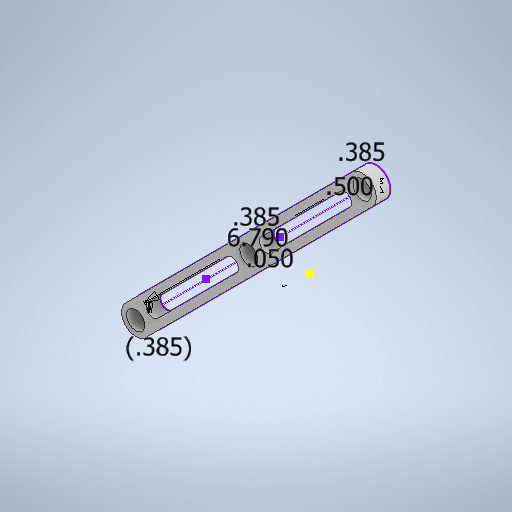
# Autodesk Inventor part: Reg Arm
Saved by Autodesk Inventor 2025.1 (Build 291241000, 241)
## iProperties
Created: 2025-10-25
Part Number: Reg Arm
Material: Generic
Document SubType Name: Modeling
Designer: benja
Density: 1 g/cm^3
Appearance: Default
Author: benja
Autodesk Inventor part; units mm, degrees
ref_plane "YZ Plane" through (0, 0, 0) normal (1, 0, 0) x (0, 1, 0)
ref_plane "XZ Plane" through (0, 0, 0) normal (0, 1, 0) x (-1, 0, 0)
ref_plane "XY Plane" through (0, 0, 0) normal (0, 0, 1) x (1, 0, 0)
sketch "Sketch1" plane through (0, 0, 0) normal (0, 0, 1) x (1, 0, 0)
  circle A0 centre (-86.3708, -61.0441) radius 4.8895
  circle A1 centre (-86.3708, -61.0441) radius 4.8895
  line L0 (-81.8807, -65.5342) -> (40.0712, 56.4176)
  line L1 (31.091, 65.3979) -> (-90.8609, -56.554)
  arc A2 (-90.8609, -56.554) -> (-81.8807, -65.5342) centre (-86.3708, -61.0441) ccw
  arc A3 (40.0712, 56.4176) -> (31.091, 65.3979) centre (35.5811, 60.9078) ccw
  circle A4 centre (-25.3948, -0.0682) radius 4.8895
  circle A5 centre (35.5811, 60.9078) radius 4.8895
  line L2 (-21.9374, 3.3892) -> (32.1237, 57.4504)
  line L3 (39.0385, 64.3652) -> (40.0712, 65.3979)
  line L4 (-82.9134, -57.5867) -> (-28.8522, -3.5256) construction
  line L5 (-21.9374, 3.3892) -> (32.1237, 57.4504) construction
  line L6 (-28.8522, -3.5256) -> (-82.9134, -57.5867)
  line L7 (-89.8282, -64.5015) -> (-90.8609, -65.5342)
  line L8 (-34.6701, -9.3434) -> (-77.0956, -51.7689) construction
  line L9 (-37.2209, -6.7925) -> (-79.6465, -49.218)
  line L10 (-74.5447, -54.3198) -> (-32.1192, -11.8943)
  arc A6 (-32.1192, -11.8943) -> (-37.2209, -6.7925) centre (-34.6701, -9.3434) ccw
  arc A7 (-79.6465, -49.218) -> (-74.5447, -54.3198) centre (-77.0956, -51.7689) ccw
  line L11 (-25.3948, -0.0682) -> (-29.885, 4.422)
  line L12 (-18.6705, 11.7579) -> (23.755, 54.1835)
  line L13 (28.8568, 49.0817) -> (-13.5688, 6.6562)
  arc A8 (-18.6705, 11.7579) -> (-13.5688, 6.6562) centre (-16.1196, 9.207) ccw
  arc A9 (28.8568, 49.0817) -> (23.755, 54.1835) centre (26.3059, 51.6326) ccw
  line L14 (40.9692, 55.5196) -> (-80.9826, -66.4323)
  arc A10 (-91.7589, -55.6559) -> (-80.9826, -66.4323) centre (-86.3708, -61.0441) ccw
  line L15 (-91.7589, -55.6559) -> (30.1929, 66.2959)
  arc A11 (40.9692, 55.5196) -> (30.1929, 66.2959) centre (35.5811, 60.9078) ccw
  point P0 (0, 0)
  point P1 (-55.8828, -30.5561)
  dimension "d0" = 172.466
  dimension "d2" = 12.7
  dimension "d5" = 9.779
  dimension "d6" = 9.779
  dimension "d7" = 9.779
  dimension "d10" = 1.27
  constraints: 34 end point, 24 point on circle, 12 centre point, 8 tangent, 6 symmetric about line, 3 midpoint, 3 parallel, 2 coincident, 1 point on line, 5 other
  measures "d0" distance of A1.centre A3.centre
  measures "d2" diameter of A3
  measures "d5" diameter of A4
  measures "d6" diameter of A1
  measures "d7" diameter of A5
  measures "d10" distance between parallel lines of L0 L14
extrude "Extrusion1" add sketch "Sketch1" along normal blind 7.62 contours A0 L6 A7 L10 A6 A4 L2 A8 L13 A9 A5 L3 A3 L0 A2 L7 | A0 L7 A2 L1 L11 A4 L6 A6 L9 A7 | L1 A3 L3 A5 L2 A9 L12 A8 A4 L11
extrude "Extrusion2" add sketch "Sketch1" along normal up to surface (7.62 mm away)
body "Solid1"
